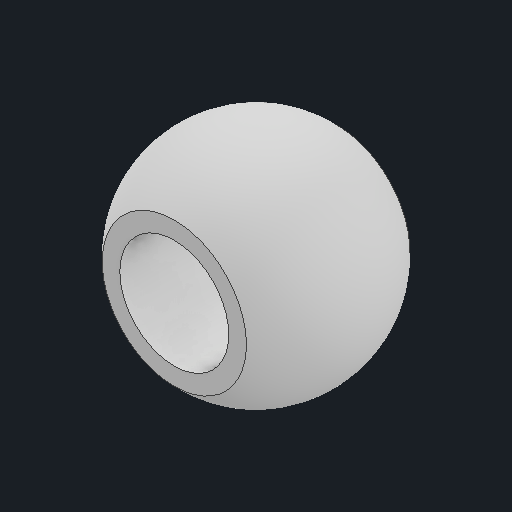
# Autodesk Inventor part: Ball_6mm_CPY_CPY
Saved by Autodesk Inventor 2023 (Build 270158000, 158)
## iProperties
Created: 2023-02-24
Part Number: Ball_6mm_CPY_CPY
Material: Generic
Document SubType Name: Modeling
Designer: roota
Density: 1 g/cm^3
Appearance: Default
Author: roota
Autodesk Inventor part; units mm, degrees
ref_plane "YZ Plane" through (0, 0, 0) normal (1, 0, 0) x (0, 1, 0)
ref_plane "XZ Plane" through (0, 0, 0) normal (0, 1, 0) x (-1, 0, 0)
ref_plane "XY Plane" through (0, 0, 0) normal (0, 0, 1) x (1, 0, 0)
sketch "Sketch1" plane through (0, 0, 0) normal (1, 0, 0) x (0, 1, 0)
  circle A0 centre (0, 0) radius 6
  line L0 (0, 6) -> (0, -6)
  line L1 (3, -5.1962) -> (3, 5.1962)
  line L2 (3.9686, 4.5) -> (3, 4.5)
  line L3 (3.9686, -4.5) -> (3, -4.5)
  dimension "d0" = 6
  dimension "d1" = 9
  dimension "d2" = 12
  constraints: 8 end point, 6 point on circle, 2 parallel, 2 perpendicular, 2 point on line, 1 centre point, 1 coincident, 1 midpoint, 1 vertical
  measures "d0" diameter of L1 L0
  measures "d1" distance between parallel lines of L2 L3
  measures "d2" diameter of A0
revolve "Revolution1" add sketch "Sketch1" angle 360 about axis through (0, 0, 6) along (0, 0, -1) contours A0 L3 L1 L2
body "Solid1"
